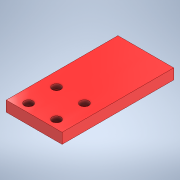
# Autodesk Inventor part: plateForPot
Saved by Autodesk Inventor 2020.2 (Build 242310000, 310)
## iProperties
Created: 2019-11-21
Part Number: plateForPot
Material: ABS Plastic
Document SubType Name: Modeling
Designer: steele
Density: 1.06 g/cm^3
Appearance: Light Red
Author: steele
Autodesk Inventor part; units mm, degrees
ref_plane "YZ Plane" through (0, 0, 0) normal (1, 0, 0) x (0, 1, 0)
ref_plane "XZ Plane" through (0, 0, 0) normal (0, 1, 0) x (-1, 0, 0)
ref_plane "XY Plane" through (0, 0, 0) normal (0, 0, 1) x (1, 0, 0)
sketch "Sketch1" plane through (0, 0, 0) normal (0, 1, 0) x (-1, 0, 0)
  line L0 (25.4, 50.8) -> (-25.4, 50.8)
  line L1 (-25.4, 50.8) -> (-25.4, -50.8)
  line L2 (-25.4, -50.8) -> (25.4, -50.8)
  line L3 (25.4, -50.8) -> (25.4, 50.8)
  line L4 (25.4, 50.8) -> (-25.4, -50.8) construction
  line L5 (-25.4, 50.8) -> (25.4, -50.8) construction
  point P0 (0, 0)
  dimension "d0" = 50.8
  dimension "d1" = 101.6
  constraints: 12 end point, 2 midpoint, 2 parallel, 1 horizontal, 1 perpendicular
  measures "d0" distance of L0.start L0.end
  measures "d1" distance of L1.end L0.end
extrude "Extrusion1" add sketch "Sketch1" along normal blind 9.525
sketch "Sketch2" plane through (0, 9.525, 0) normal (0, 1, 0) x (1, 0, 0)
  line L0 (-12.7, -43.18) -> (12.7, -43.18) construction
  line L1 (12.7, -43.18) -> (12.7, -17.78) construction
  line L2 (12.7, -17.78) -> (-12.7, -17.78) construction
  line L3 (-12.7, -17.78) -> (-12.7, -43.18) construction
  line L4 (-12.7, -43.18) -> (12.7, -17.78) construction
  line L5 (12.7, -43.18) -> (-12.7, -17.78) construction
  line L6 (-25.4, -50.8) -> (25.4, -50.8) projected
  point P0 (0, 0)
  point P1 (0, -30.48)
  dimension "d4" = 25.4
  dimension "d5" = 25.4
  dimension "d6" = 7.62
  constraints: 12 end point, 4 coincident, 2 midpoint, 2 parallel, 1 horizontal, 1 perpendicular
  measures "d4" distance of L0.start L0.end
  measures "d5" distance of L1.end L0.end
  measures "d6" distance between parallel lines of L0 L6
hole "Hole1" at (-12.7, 9.525, 43.18) at (12.7, 9.525, 43.18) at (12.7, 9.525, 17.78) at (-12.7, 9.525, 17.78) direction (0, -1, 0) diameter 4.4958 end through all counterbore diameter 7.9502 counterbore depth 4.1656 clearance for "Socket Head Cap Screw" size "#8" standard "Ansi Unified Screw Threads"
body "Solid1"
